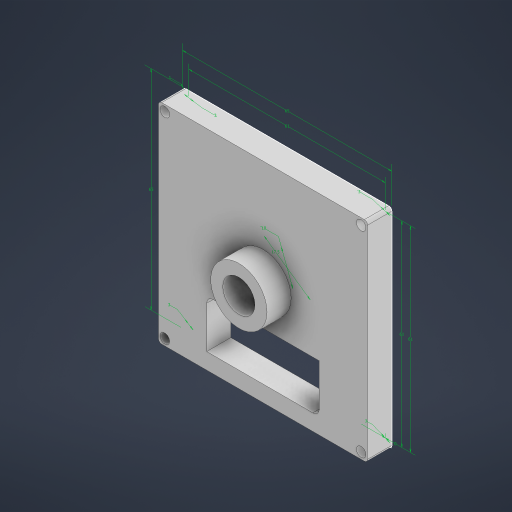
# Autodesk Inventor part: top
Saved by Autodesk Inventor 2023 (Build 270158000, 158)
## iProperties
Created: 2022-11-09
Part Number: top
Material: Generic
Document SubType Name: Modeling
Designer: Mike
Density: 1 g/cm^3
Appearance: Default
Author: Mike
Autodesk Inventor part; units mm, degrees
ref_plane "YZ Plane" through (0, 0, 0) normal (1, 0, 0) x (0, 1, 0)
ref_plane "XZ Plane" through (0, 0, 0) normal (0, 1, 0) x (-1, 0, 0)
ref_plane "XY Plane" through (0, 0, 0) normal (0, 0, 1) x (1, 0, 0)
sketch "Sketch1" plane through (0, 0, 0) normal (0, 0, 1) x (1, 0, 0)
  line L0 (-30.5, -30.5) -> (30.5, -30.5) construction
  line L1 (30.5, -30.5) -> (30.5, 30.5) construction
  line L2 (30.5, 30.5) -> (-30.5, 30.5) construction
  line L3 (-30.5, 30.5) -> (-30.5, -30.5) construction
  line L4 (-30.5, -30.5) -> (30.5, 30.5) construction
  line L5 (30.5, -30.5) -> (-30.5, 30.5) construction
  circle A0 centre (0, 0) radius 5
  circle A1 centre (-30.5, 30.5) radius 1.5
  circle A2 centre (30.5, 30.5) radius 1.5
  circle A3 centre (-30.5, -30.5) radius 1.5
  circle A4 centre (30.5, -30.5) radius 1.5
  line L6 (31.5, -32.5) -> (-31.5, -32.5)
  line L7 (-32.5, -31.5) -> (-32.5, 31.5)
  line L8 (-31.5, 32.5) -> (31.5, 32.5)
  line L9 (32.5, 31.5) -> (32.5, -31.5)
  line L10 (32.5, -32.5) -> (-32.5, 32.5) construction
  line L11 (-32.5, -32.5) -> (32.5, 32.5) construction
  arc A5 (-31.5, 32.5) -> (-32.5, 31.5) centre (-31.5, 31.5) ccw
  arc A6 (32.5, 31.5) -> (31.5, 32.5) centre (31.5, 31.5) ccw
  arc A7 (31.5, -32.5) -> (32.5, -31.5) centre (31.5, -31.5) ccw
  arc A8 (-32.5, -31.5) -> (-31.5, -32.5) centre (-31.5, -31.5) ccw
  circle A9 centre (0, 0) radius 8.75
  dimension "d0" = 61
  dimension "d1" = 61
  dimension "d2" = 10
  dimension "d3" = 3
  dimension "d4" = 3
  dimension "d5" = 3
  dimension "d6" = 3
  dimension "d7" = 0
  dimension "d8" = 61
  dimension "d9" = 65
  dimension "d10" = 65
  dimension "d11" = 1
  dimension "d12" = 17.5
  constraints: 24 end point, 10 centre point, 8 point on circle, 8 point on line, 8 tangent, 5 coincident, 4 midpoint, 4 parallel, 3 equal radius, 2 horizontal, 2 perpendicular
  measures "d0" distance of L2.end L1.end
  measures "d1" distance of L1.end L0.end
  measures "d2" diameter of A0
  measures "d3" diameter of A1
  measures "d4" diameter of A2
  measures "d5" diameter of A3
  measures "d6" diameter of A4
  measures "d7" distance from line of A4.centre L1
  measures "d8" distance from line of A4.centre L2
  measures "d9" distance of L10.end L11.end
  measures "d10" distance of L11.start L10.end
  measures "d11" radius of A5
  measures "d12" diameter of A9
extrude "Extrusion1" add sketch "Sketch1" along normal blind 7.5 contours L6 A8 L7 A5 L8 A6 L9 A7
extrude "Extrusion2" add sketch "Sketch1" along normal blind 15 contours A9
sketch "Sketch2" plane through (0, 0, 7.5) normal (0, 0, 1) x (1, 0, 0)
  line L0 (-15.5, -12.5) -> (17.5, -12.5)
  line L1 (17.5, -12.5) -> (17.5, -25.5)
  line L2 (15.5, -27.5) -> (-17.5, -27.5)
  line L3 (-17.5, -27.5) -> (-17.5, -14.5)
  line L4 (-32.5, 31.5) -> (-32.5, -31.5) projected
  line L5 (32.5, -31.5) -> (32.5, 31.5) projected
  line L6 (-31.5, -32.5) -> (31.5, -32.5) projected
  arc A0 (-15.5, -12.5) -> (-17.5, -14.5) centre (-15.5, -14.5) ccw
  arc A1 (15.5, -27.5) -> (17.5, -25.5) centre (15.5, -25.5) ccw
  point P0 (0, 0)
  dimension "d17" = 15
  dimension "d18" = 15
  dimension "d19" = 5
  dimension "d20" = 15
  dimension "d21" = 2
  constraints: 8 end point, 4 point on circle, 4 tangent, 2 centre point, 2 parallel, 1 equal radius, 1 horizontal, 1 perpendicular
  measures "d17" distance between parallel lines of L4 L3
  measures "d18" distance between parallel lines of L5 L1
  measures "d19" distance between parallel lines of L6 L2
  measures "d20" distance between parallel lines of L2 L0
  measures "d21" radius of A0
extrude "Extrusion3" cut sketch "Sketch2" against normal up to surface (7.5 mm away)
body "Solid1"
